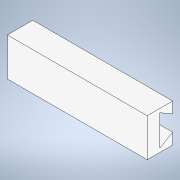
# Autodesk Inventor part: Runway
Saved by Autodesk Inventor 2020.5 (Build 245400000, 400)
## iProperties
Created: 2020-02-29
Part Number: Runway
Document SubType Name: Modeling
Designer: Administrator
Density: 7.85 g/cm^3
Material: Acero, carbono
Appearance: White
Mass: 1.69594 g
Surface Area: 10.4838 cm^2
Volume: 1.69594 cm^3
Author: Administrator
Autodesk Inventor part; units mm, degrees
ref_plane "YZ Plane" through (0, 0, 0) normal (1, 0, 0) x (0, 1, 0)
ref_plane "XZ Plane" through (0, 0, 0) normal (0, 1, 0) x (-1, 0, 0)
ref_plane "XY Plane" through (0, 0, 0) normal (0, 0, 1) x (1, 0, 0)
sketch "Sketch4" plane through (0, 0, 0) normal (1, 0, 0) x (0, 1, 0)
  line L0 (0, 0) -> (0, -12)
  line L1 (0, -12) -> (10, -6.2265)
  line L2 (10, -6.2265) -> (10, 6.2265) construction
  line L3 (10, 6.2265) -> (0, 12)
  line L4 (0, 12) -> (0, 0)
  line L5 (0, 0) -> (10, 0) construction
  line L6 (10, 6.2265) -> (10, 15)
  line L7 (10, 15) -> (-10, 15)
  line L8 (-10, 15) -> (-10, -15)
  line L9 (-10, -15) -> (10, -15)
  line L10 (10, -15) -> (10, -6.2265)
  dimension "d31" = 60
  dimension "d32" = 60
  dimension "d33" = 10
  dimension "d34" = 12
  dimension "d43" = 10
  dimension "d44" = 30
  constraints: 22 end point, 3 collinear, 3 parallel, 3 perpendicular, 3 point on line, 1 midpoint, 1 vertical
  measures "d31" angle of L0 L1
  measures "d32" angle of L4 L3
  measures "d33" distance between parallel lines of L2 L0
  measures "d34" distance of L0.start L0.end
  measures "d44" distance of L7.end L8.end
extrude "Extrusion3" add sketch "Sketch4" along normal mid plane 110
body "Solid4"
